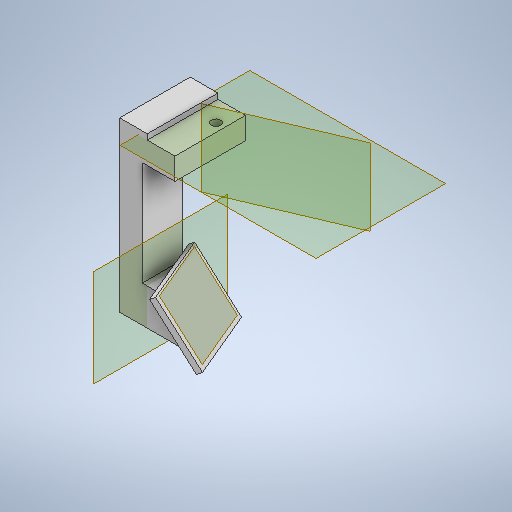
# Autodesk Inventor part: uchwycik_lustra
Saved by Autodesk Inventor 2025.1 (Build 291241000, 241)
## iProperties
Created: 2024-10-13
Part Number: uchwycik_lustra
Material: Ogólny
Document SubType Name: Modeling
Designer: zychlix
Density: 1 g/cm^3
Appearance: Domyślna
Author: zychlix
Autodesk Inventor part; units mm, degrees
ref_plane "YZ Plane" through (0, 0, 0) normal (1, 0, 0) x (0, 1, 0)
ref_plane "XZ Plane" through (0, 0, 0) normal (0, 1, 0) x (-1, 0, 0)
ref_plane "Płaszczyzna konstrukcyjna1" through (-54.9466, -54.6295, -13.1077) normal (-0.7718631, -0.544639, 0.3280178) x (-0.3886148, -0.0041773, -0.9213908)
sketch "Szkic2" plane through (-54.9466, -54.6295, -13.1077) normal (-0.7718631, -0.544639, 0.3280178) x (-0.3886148, -0.0041773, -0.9213908)
  line L0 (13.042, -11.6942) -> (-13.7093, -11.6942)
  line L1 (-13.7093, -11.6942) -> (-13.7093, 12.3632)
  line L2 (-13.7093, 12.3632) -> (13.042, 12.3632)
  line L3 (13.042, 12.3632) -> (13.042, -11.6942)
  point P0 (-33.6586, -20.8987)
  constraints: 8 end point, 2 parallel, 1 horizontal, 1 perpendicular
extrude "Wyciągnięcie proste1" add sketch "Szkic2" along normal blind 2
ref_plane "Płaszczyzna konstrukcyjna2" through (-32.4801, 0, -22.4835) normal (-0.3911164, 0, -0.9203412) x (-0.9203412, 0, 0.3911164)
ref_plane "Płaszczyzna konstrukcyjna3" through (-65, -3, 0) normal (-1, 0, 0) x (0, 0, 1)
sketch "Szkic4" plane through (-65, -3, 0) normal (-1, 0, 0) x (0, 0, 1)
  line L0 (-19.3072, -59.4209) -> (-4.4436, -59.4209)
  line L1 (-4.4436, -59.4209) -> (-4.4436, -46.1044)
  line L2 (-4.4436, -46.1044) -> (-19.3072, -46.1044)
  line L3 (-19.3072, -46.1044) -> (-19.3072, -59.4209)
  point P0 (0, 3)
  constraints: 8 end point, 2 parallel, 1 horizontal, 1 perpendicular
extrude "Wyciągnięcie proste2" add sketch "Szkic4" along normal up to surface surface through (-56.1924, -55.9979, -12.214) normal (-0.7718631, -0.544639, 0.3280178)
sketch "Szkic5" plane through (-65, -3, 0) normal (-1, 0, 0) x (0, 0, 1)
  line L0 (-4.4436, -59.4209) -> (-4.4436, -46.1044) projected
  line L1 (-4.4436, -46.1044) -> (-19.3072, -46.1044) projected
  line L2 (-19.3072, -46.1044) -> (-19.3072, -59.4209) projected
  line L3 (-19.3072, -59.4209) -> (-4.4436, -59.4209) projected
  line L4 (0, 0) -> (-41, 0) projected
  line L5 (-4.4436, -59.4209) -> (-4.4436, -46.1044) projected
  line L6 (-4.4436, -59.4209) -> (-19.3072, -59.4209)
  line L7 (-19.3072, -59.4209) -> (-19.3072, 0)
  line L8 (-19.3072, 0) -> (-4.4436, 0)
  line L9 (-4.4436, 0) -> (-4.4436, -59.4209)
  line L10 (-4.4436, -46.1044) -> (-19.3072, -46.1044)
  point P0 (0, 3)
  constraints: 10 end point, 3 equal length, 1 horizontal, 1 perpendicular, 1 point on line
extrude "Wyciągnięcie proste3" add sketch "Szkic5" along normal blind 10 contours L3 L2 L1 L0
sketch "Szkic6" plane through (-75, -49.1044, -4.4436) normal (0, 1, 0) x (1, 0, 0)
  line L0 (0, 0) -> (0, 14.8637) projected
  line L1 (0, 14.8637) -> (8.2365, 14.8637)
  line L2 (8.2365, 14.8637) -> (8.2365, 0)
  line L3 (8.2365, 0) -> (0, 0)
  line L4 (0, 0) -> (0, 14.8637)
  line L5 (10, -4.4436) -> (10, 36.5564)
  line L6 (0, 14.8637) -> (10, 14.8637)
  line L7 (10, 14.8637) -> (10, 0)
  line L8 (10, 0) -> (0, 0)
  line L9 (0, 0) -> (0, 14.8637)
  point P0 (75, -4.4436)
  constraints: 18 end point, 4 parallel, 2 horizontal, 2 perpendicular, 1 point on line, 1 vertical, 2 other
ref_plane "Płaszczyzna konstrukcyjna4" through (-65, -3, -43) normal (0, -1, 0) x (1, 0, 0)
extrude "Wyciągnięcie proste4" add sketch "Szkic6" along normal up to surface (46.1044 mm away) contours L0 L1 L2 L3
ref_plane "Płaszczyzna konstrukcyjna5" through (-32.5, -3, -21.5) normal (0, -1, 0) x (-1, 0, 0)
sketch "Szkic7" plane through (-32.5, -3, -21.5) normal (0, -1, 0) x (-1, 0, 0)
  line L0 (42.5, -17.0564) -> (34.2635, -17.0564) projected
  line L1 (42.5, -17.0564) -> (22.3226, -17.0564)
  line L2 (22.3226, -17.0564) -> (22.3226, 8.7067)
  line L3 (22.3226, 8.7067) -> (42.5, 8.7067)
  line L4 (42.5, 8.7067) -> (42.5, -17.0564)
  circle A0 centre (25.3725, 0.975) radius 1.45 projected
  circle A1 centre (25.3725, 0.975) radius 1.7
  point P0 (-32.5, -21.5)
  point P1 (34.2635, -17.0564)
  dimension "d10" = 3.4
  constraints: 8 end point, 2 parallel, 1 centre point, 1 coincident, 1 horizontal, 1 perpendicular
  measures "d10" diameter of A1
extrude "Wyciągnięcie proste5" add sketch "Szkic7" along normal blind 8 contours L0 L1 L2 L3 L4
sketch "Szkic8" plane through (-75, -3, -30.2067) normal (0, 1, 0) x (1, 0, 0)
  line L0 (0, 0) -> (0, -25.7631) projected
  line L1 (0, -25.7631) -> (20.1774, -25.7631) projected
  line L2 (0, 0) -> (10.0887, 0)
  line L3 (10.0887, 0) -> (10.0887, -25.7631)
  line L4 (10.0887, -25.7631) -> (0, -25.7631)
  line L5 (0, -25.7631) -> (0, 0)
  point P0 (75, -30.2067)
  constraints: 8 end point, 2 parallel, 1 horizontal, 1 midpoint, 1 perpendicular
extrude "Wyciągnięcie proste6" add sketch "Szkic8" along normal blind 2
